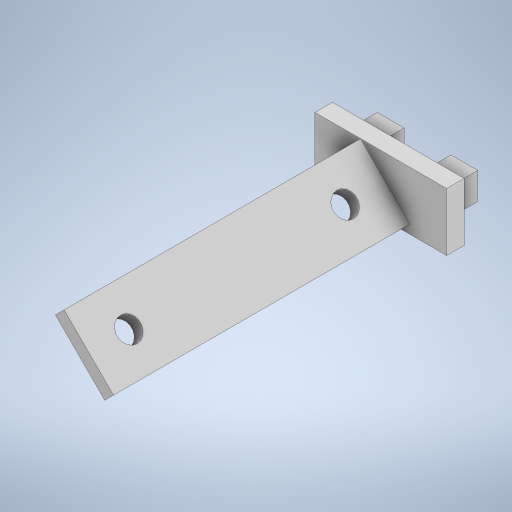
# Autodesk Inventor part: IR45
Saved by Autodesk Inventor 2024 (Build 280153000, 153)
## iProperties
Created: 2024-05-03
Part Number: IR45
Material: Generic
Document SubType Name: Modeling
Designer: cyan924
Density: 1 g/cm^3
Appearance: Default
Author: cyan924
Autodesk Inventor part; units mm, degrees
ref_plane "YZ Plane" through (0, 0, 0) normal (1, 0, 0) x (0, 1, 0)
ref_plane "XZ Plane" through (0, 0, 0) normal (0, 1, 0) x (-1, 0, 0)
ref_plane "XY Plane" through (0, 0, 0) normal (0, 0, 1) x (1, 0, 0)
sketch "Sketch1" plane through (0, 0, 0) normal (0, 0, 1) x (1, 0, 0)
  line L0 (0, 0) -> (4.6, 0)
  line L1 (4.6, 0) -> (4.6, 4.6)
  line L2 (4.6, 4.6) -> (0, 4.6)
  line L3 (0, 4.6) -> (0, 0)
  line L4 (4.6, 4.6) -> (12.6, 4.6) construction
  line L5 (12.6, 4.6) -> (17.2, 4.6)
  line L6 (17.2, 4.6) -> (17.2, 0)
  line L7 (17.2, 0) -> (12.6, 0)
  line L8 (12.6, 0) -> (12.6, 4.6)
  dimension "d2" = 4.6
  dimension "d3" = 4.6
  dimension "d4" = 8
  dimension "d5" = 4.6
  constraints: 18 end point, 4 parallel, 3 horizontal, 2 perpendicular
  measures "d2" distance of L2.end L1.end
  measures "d3" distance of L1.end L0.end
  measures "d4" distance of L1.end L4.end
  measures "d5" distance of L6.end L7.end
extrude "Extrusion1" add sketch "Sketch1" along normal blind 5
sketch "Sketch2" plane through (0, 0, 5) normal (0, 0, 1) x (1, 0, 0)
  line L0 (17.2, 0) -> (17.2, -2.6667) construction
  line L1 (17.2, -2.6667) -> (19.8667, -2.6667) construction
  line L2 (0, 4.6) -> (0, 7.2667) construction
  line L3 (0, 7.2667) -> (-2.6667, 7.2667) construction
  line L4 (-2.6667, 7.2667) -> (19.8667, 7.2667)
  line L5 (19.8667, 7.2667) -> (19.8667, -2.6667)
  line L6 (19.8667, -2.6667) -> (-2.6667, -2.6667)
  line L7 (-2.6667, -2.6667) -> (-2.6667, 7.2667)
  point P0 (29.8, 0)
  dimension "d18" = 2.6667
  dimension "d19" = 2.6667
  dimension "d20" = 2.6667
  dimension "d21" = 2.6667
  constraints: 16 end point, 3 perpendicular, 2 parallel, 2 vertical, 1 horizontal
  measures "d18" distance of L0.start L0.end
  measures "d19" distance of L0.end L1.end
  measures "d20" distance of L2.start L2.end
  measures "d21" distance of L2.end L3.end
extrude "Extrusion2" add sketch "Sketch2" along normal blind 3
sketch "Sketch3" plane through (0, 0, 8) normal (0, 0, 1) x (1, 0, 0)
  line L0 (19.8667, -2.6667) -> (19.8667, 7.2667) construction
  line L1 (19.8667, 7.2667) -> (-2.6667, 7.2667) construction
  line L2 (-2.6667, -2.6667) -> (19.8667, -2.6667) construction
  line L3 (-2.6667, 7.2667) -> (-2.6667, -2.6667) construction
  line L4 (-2.6667, 2.3) -> (19.8667, 2.3) construction
  line L5 (8.6, 7.2667) -> (8.6, -2.6667) construction
  line L6 (8.6, 2.3) -> (7.85, 3.05) construction
  line L7 (8.6, 2.3) -> (9.35, 1.55) construction
  line L8 (8.6, 2.3) -> (9.35, 3.05) construction
  line L9 (8.6, 2.3) -> (7.85, 1.55) construction
  line L10 (9.35, 3.05) -> (5.1333, 7.2667)
  line L11 (7.85, 1.55) -> (12.0667, -2.6667)
  line L12 (9.35, 3.05) -> (13.5667, -1.1667)
  line L13 (13.5667, -1.1667) -> (12.0667, -2.6667)
  line L14 (7.85, 1.55) -> (3.6333, 5.7667)
  line L15 (3.6333, 5.7667) -> (5.1333, 7.2667)
  point P0 (0, 0)
  dimension "d46" = 0.75
  dimension "d47" = 45
  dimension "d48" = 45
  dimension "d49" = 0.75
  constraints: 24 end point, 5 midpoint, 3 perpendicular, 3 point on line, 1 parallel
  measures "d46" distance from line of L4 L8.end
  measures "d47" angle of L4 L8
  measures "d48" angle of L5 L9
  measures "d49" distance from line of L4 L9.end
extrude "Extrusion4" add sketch "Sketch3" along normal blind 50.7
sketch "Sketch5" plane through (5.1333, 7.2667, 8) normal (0.7071, 0.7071, 0) x (-0.7071, 0.7071, 0)
  line L0 (0, 0.0299) -> (-11.9265, -0.0248) construction
  line L1 (-5.9633, 0.0025) -> (-5.9633, 50.7) construction
  line L2 (0, 50.7) -> (-10.418, 50.7) construction
  line L3 (-11.9265, 50.7547) -> (-11.9265, -0.0248) construction
  line L4 (-11.9265, 25.3649) -> (0, 25.3649) construction
  line L5 (0, 50.7) -> (0, 0.0299) construction
  line L6 (-5.9633, 25.3649) -> (-5.9633, 6.8649) construction
  line L7 (-5.9633, 25.3649) -> (-5.9633, 43.8649) construction
  circle A0 centre (-5.9633, 6.8649) radius 2
  circle A1 centre (-5.9633, 43.8649) radius 2
  line L8 (-11.9265, 0) -> (-11.9265, 50.7) projected
  line L9 (-11.9265, 50.7) -> (0, 50.7) projected
  point P0 (-1.5085, -8)
  point P1 (5.5376, 58.6752)
  dimension "d50" = 18.5
  dimension "d51" = 18.5
  dimension "d52" = 4
  dimension "d53" = 4
  dimension "d54" = 0
  dimension "d55" = 0
  constraints: 16 end point, 4 midpoint, 3 point on line, 2 centre point, 2 coincident, 1 collinear, 1 perpendicular, 1 vertical
  measures "d50" distance of L6.start L6.end
  measures "d51" distance of L6.start L7.end
  measures "d52" diameter of A0
  measures "d53" diameter of A1
  measures "d54" distance between parallel lines of L8 L3
  measures "d55" distance between parallel lines of L9 L2
extrude "Extrusion6" cut sketch "Sketch5" against normal blind 50.7
equation "\"d2\" = box"
equation "\"d3\" = box"
equation "\"d4\" = gap"
equation "\"d5\" = box"
equation "\"d18\" = 0.333333 * gap"
equation "\"d19\" = 0.333333 * gap"
equation "\"d20\" = 0.333333 * gap"
equation "\"d21\" = 0.333333 * gap"
equation "\"box\" = 4.6"
equation "\"gap\" = 8"
body "Solid1"
